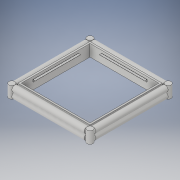
# Autodesk Inventor part: bumpers
Saved by Autodesk Inventor 2018 (Build 220112000, 112)
## iProperties
Created: 2019-02-23
Part Number: bumpers
Material: Generic
Document SubType Name: Modeling
Designer: s-2513226
Density: 1 g/cm^3
Appearance: Default
Author: s-2513226
Autodesk Inventor part; units mm, degrees
ref_plane "YZ Plane" through (0, 0, 0) normal (1, 0, 0) x (0, 1, 0)
ref_plane "XZ Plane" through (0, 0, 0) normal (0, 1, 0) x (-1, 0, 0)
ref_plane "XY Plane" through (0, 0, 0) normal (0, 0, 1) x (1, 0, 0)
sketch "Sketch1" plane through (0, 0, 0) normal (0, 0, 1) x (1, 0, 0)
  line L0 (0, 0) -> (-18.923, 0)
  line L1 (-18.923, 0) -> (-18.923, -127)
  line L2 (-18.923, -127) -> (0, -127)
  line L3 (0, -127) -> (0, 0)
  dimension "d0" = 127
  dimension "d1" = 18.923
  constraints: 8 end point, 2 parallel, 1 horizontal, 1 perpendicular
  measures "d0" distance of L0.end L1.end
  measures "d1" distance of L1.end L2.end
extrude "Extrusion1" add sketch "Sketch1" along normal blind 762
sketch "Sketch2" plane through (0, -127, 0) normal (1, 0, 0) x (0, 0, -1)
  line L0 (0, 127) -> (0, 0) projected
  line L1 (0, 127) -> (-18.923, 127)
  line L2 (-18.923, 127) -> (-18.923, 0)
  line L3 (-18.923, 0) -> (0, 0)
  line L4 (0, 0) -> (0, 127)
  dimension "d4" = 18.923
  dimension "d21" = 127
  constraints: 8 end point, 2 parallel, 1 horizontal, 1 perpendicular
  measures "d4" distance of L0.start L1.end
  measures "d21" distance of L3.end L0.start
extrude "Extrusion2" add sketch "Sketch2" along normal blind 762
sketch "Sketch3" plane through (0, -139.7, 18.923) normal (0, 0, 1) x (1, 0, 0)
  line L0 (762, 139.7) -> (-18.923, 139.7) projected
  line L1 (762, 139.7) -> (743.077, 139.7)
  line L2 (743.077, 139.7) -> (743.077, 12.7)
  line L3 (743.077, 12.7) -> (762, 12.7)
  line L4 (762, 12.7) -> (762, 139.7)
  line L5 (0, 12.7) -> (762, 12.7) projected
  point P0 (0, 139.7)
  dimension "d8" = 18.923
  constraints: 8 end point, 2 parallel, 1 horizontal, 1 perpendicular
  measures "d8" distance of L2.end L3.end
extrude "Extrusion3" add sketch "Sketch3" along normal blind 762
sketch "Sketch4" plane through (743.077, -127, 18.923) normal (-1, 0, 0) x (0, 0, 1)
  line L0 (762, 0) -> (762, 127) projected
  line L1 (762, 127) -> (743.077, 127)
  line L2 (743.077, 127) -> (743.077, 0)
  line L3 (743.077, 0) -> (762, 0)
  line L4 (762, 0) -> (762, 127)
  line L5 (0, 0) -> (762, 0) projected
  point P0 (-18.923, 127)
  dimension "d11" = 18.923
  dimension "d12" = 0
  constraints: 8 end point, 2 parallel, 1 horizontal, 1 perpendicular
  measures "d11" distance of L0.end L1.end
  measures "d12" distance between parallel lines of L5 L3
extrude "Extrusion4" add sketch "Sketch4" along normal blind 762
sketch "Sketch8" plane through (0, -139.7, 780.923) normal (0, 0, 1) x (1, 0, 0)
  circle A0 centre (-50.673, 107.95) radius 31.75
  circle A1 centre (-50.673, 44.45) radius 31.75
  line L0 (762, 12.7) -> (-18.923, 12.7) projected
  line L1 (762, 139.7) -> (-18.923, 139.7) projected
  line L2 (-18.923, 12.7) -> (-18.923, 139.7) projected
  point P0 (0, 139.7)
  dimension "d32" = 63.5
  dimension "d33" = 63.5
  dimension "d35" = 31.75
  dimension "d36" = 31.75
  dimension "d37" = 31.75
  dimension "d38" = 31.75
  constraints: 2 centre point
  measures "d32" diameter of A0
  measures "d33" diameter of A1
  measures "d35" distance from line of L1 A0.centre
  measures "d36" distance from line of L0 A1.centre
  measures "d37" distance from line of L2 A1.centre
  measures "d38" distance from line of L2 A0.centre
extrude "Extrusion7" add sketch "Sketch8" against normal blind 780.923 contours A0 | A1
sketch "Sketch10" plane through (-18.923, 0, 0) normal (-1, 0, 0) x (0, 0, 1)
  circle A0 centre (-31.75, -31.75) radius 31.75
  circle A1 centre (-31.75, -95.25) radius 31.75
  line L0 (0, 0) -> (0, -31.75) projected
  line L1 (0, 0) -> (780.923, 0) projected
  line L2 (0, 0) -> (0, -31.75) projected
  point P0 (0, -127)
  point P1 (0, -95.25)
  dimension "d41" = 63.5
  dimension "d42" = 63.5
  dimension "d43" = 31.75
  dimension "d44" = 31.75
  dimension "d45" = 31.75
  dimension "d46" = 31.75
  dimension "d47" = 31.75
  constraints: 2 centre point
  measures "d41" diameter of A0
  measures "d42" diameter of A1
  measures "d43" horizontal distance of point (0, -127) A1.centre
  measures "d44" horizontal distance of L0.start A0.centre
  measures "d45" distance from line of L0 A0.centre
  measures "d46" distance from line of L1 A0.centre
  measures "d47" distance from line of L2 A1.centre
extrude "Extrusion8" add sketch "Sketch10" against normal blind 780.923
sketch "Sketch12" plane through (0, 0, 0) normal (0, 0, -1) x (-1, 0, 0)
  circle A0 centre (-793.75, -31.75) radius 31.75
  circle A1 centre (-793.75, -95.25) radius 31.75
  line L0 (-762, -63.5) -> (-762, -127) projected
  line L1 (-762, 0) -> (-762, -63.5) projected
  line L2 (-762, 0) -> (18.923, 0) projected
  line L3 (18.923, -127) -> (-762, -127) projected
  point P0 (0, 0)
  point P1 (-762, -95.25)
  point P2 (-762, -31.75)
  dimension "d50" = 63.5
  dimension "d51" = 63.5
  dimension "d52" = 31.75
  dimension "d53" = 31.75
  dimension "d54" = 31.75
  dimension "d55" = 31.75
  constraints: 2 centre point
  measures "d50" diameter of A0
  measures "d51" diameter of A1
  measures "d52" distance from line of L0 A1.centre
  measures "d53" distance from line of L1 A0.centre
  measures "d54" distance from line of L2 A0.centre
  measures "d55" distance from line of L3 A1.centre
extrude "Extrusion9" add sketch "Sketch12" against normal blind 780.923 contours A0 | A1
sketch "Sketch13" plane through (762, -127, 0) normal (1, 0, 0) x (0, 0, -1)
  circle A0 centre (-812.673, 95.25) radius 31.75
  circle A1 centre (-812.673, 31.75) radius 31.75
  line L0 (0, 127) -> (-780.923, 127) projected
  line L1 (-780.923, 127) -> (-780.923, 63.5) projected
  line L2 (-780.923, 63.5) -> (-780.923, 0) projected
  point P0 (0, 0)
  point P1 (-762, -95.25)
  point P2 (-762, -31.75)
  point P3 (-780.923, 95.25)
  point P4 (-780.923, 31.75)
  dimension "d58" = 63.5
  dimension "d59" = 63.5
  dimension "d64" = 63.5
  dimension "d65" = 31.75
  dimension "d66" = 31.75
  dimension "d67" = 31.75
  constraints: 2 centre point
  measures "d58" diameter of A0
  measures "d59" diameter of A1
  measures "d64" distance of A1.centre A0.centre
  measures "d65" distance from line of L0 A0.centre
  measures "d66" distance from line of L1 A0.centre
  measures "d67" distance from line of L2 A1.centre
extrude "Extrusion10" add sketch "Sketch13" against normal blind 780.923 contours A0 | A1
sketch "Sketch14" plane through (-18.923, 0, 0) normal (0, 1, 0) x (1, 0, 0)
  line L0 (780.923, 0) -> (812.673, 0) projected
  circle A0 centre (812.673, 31.75) radius 31.75
  line L1 (780.923, 0) -> (844.423, 0) projected
  line L2 (780.923, 0) -> (780.923, 63.5) projected
  circle A1 centre (-31.75, 31.75) radius 31.75
  line L3 (0, 0) -> (0, 63.5) projected
  line L4 (0, 0) -> (-63.5, 0) projected
  circle A2 centre (-31.75, -812.673) radius 31.75
  line L5 (0, -780.923) -> (-63.5, -780.923) projected
  line L6 (0, -780.923) -> (0, -844.423) projected
  circle A3 centre (812.673, -812.673) radius 31.75
  line L7 (780.923, -780.923) -> (844.423, -780.923) projected
  line L8 (780.923, -780.923) -> (780.923, -844.423) projected
  point P0 (18.923, 0)
  point P1 (780.923, 31.75)
  point P2 (0, 31.75)
  point P3 (-31.75, 0)
  point P4 (-31.75, -780.923)
  point P5 (0, -812.673)
  point P6 (812.673, -780.923)
  point P7 (780.923, -812.673)
  dimension "d73" = 63.5
  dimension "d76" = 63.5
  dimension "d70" = 31.75
  dimension "d71" = 63.5
  dimension "d72" = 31.75
  dimension "d74" = 31.75
  dimension "d75" = 31.75
  dimension "d77" = 31.75
  dimension "d78" = 31.75
  dimension "d79" = 63.5
  dimension "d80" = 31.75
  dimension "d81" = 31.75
  constraints: 2 centre point, 1 horizontal alignment, 1 point on circle, 1 vertical alignment, 2 other
  measures "d70" distance from line of L1 A0.centre
  measures "d71" diameter of A0
  measures "d72" distance from line of L2 A0.centre
  measures "d74" distance from line of point (-31.75, 31.75) L3
  measures "d75" distance from line of L4 point (-31.75, 31.75)
  measures "d77" distance from line of L5 point (-31.75, -812.673)
  measures "d78" distance from line of point (-31.75, -812.673) L6
  measures "d79" diameter of A3
  measures "d80" distance from line of L7 A3.centre
  measures "d81" distance from line of L8 A3.centre
extrude "Extrusion11" add sketch "Sketch14" against normal blind 127 contours A0 | A1 | A2 | A3
sketch "Sketch15" plane through (0, -127, 18.923) normal (1, 0, 0) x (0, 0, -1)
  line L0 (0, 0) -> (0, 127) projected
  line L1 (-743.077, 0) -> (-743.077, 127) projected
  line L2 (0, 0) -> (-743.077, 0) projected
  line L3 (18.923, 0) -> (-762, 0) projected
  line L4 (-616.077, 73.66) -> (-127, 73.66)
  line L5 (-127, 73.66) -> (-127, 99.06)
  line L6 (-127, 99.06) -> (-616.077, 99.06)
  line L7 (-616.077, 99.06) -> (-616.077, 73.66)
  point P0 (18.923, 127)
  point P1 (-127, 0)
  point P2 (-590.677, 0)
  point P3 (-152.4, 0)
  point P4 (-336.677, 0)
  point P5 (-762, 0)
  dimension "d99" = 25.4
  dimension "d100" = 73.66
  dimension "d101" = 127
  dimension "d102" = 127
  constraints: 8 end point, 2 parallel, 1 horizontal, 1 perpendicular, 4 other
  measures "d99" distance of L6.end L4.start
  measures "d100" distance of the line from the sketch origin of L4
  measures "d101" distance between parallel lines of L1 L7
  measures "d102" distance between parallel lines of L0 L5
extrude "Extrusion15" add sketch "Sketch15" along normal blind 1.651
sketch "Sketch17" plane through (1.651, -127, 18.923) normal (1, 0, 0) x (0, 0, -1)
  line L0 (-127, 99.06) -> (-616.077, 99.06) projected
  line L1 (-127, 99.06) -> (-127, 73.66) projected
  line L2 (-616.077, 99.06) -> (-127, 99.06)
  line L3 (-127, 99.06) -> (-127, 97.409)
  line L4 (-127, 97.409) -> (-616.077, 97.409)
  line L5 (-616.077, 97.409) -> (-616.077, 99.06)
  point P0 (18.923, 127)
  dimension "d105" = 1.651
  constraints: 8 end point, 2 parallel, 1 horizontal, 1 perpendicular, 1 point on line
  measures "d105" distance of L2.end L3.end
extrude "Extrusion16" add sketch "Sketch17" along normal blind 23.749
sketch "Sketch20" plane through (743.077, -127, 762) normal (0, 0, -1) x (-1, 0, 0)
  line L0 (127, 73.66) -> (616.077, 73.66)
  line L1 (616.077, 73.66) -> (616.077, 99.06)
  line L2 (616.077, 99.06) -> (127, 99.06)
  line L3 (127, 99.06) -> (127, 73.66)
  line L4 (0, 0) -> (743.077, 0) projected
  line L5 (743.077, 0) -> (743.077, 127) projected
  line L6 (0, 0) -> (0, 127) projected
  dimension "d115" = 25.4
  dimension "d116" = 73.66
  dimension "d117" = 127
  dimension "d118" = 489.077
  dimension "d119" = 127
  constraints: 8 end point, 2 parallel, 1 horizontal, 1 perpendicular
  measures "d115" distance of L2.end L0.start
  measures "d116" distance between parallel lines of L4 L0
  measures "d117" distance between parallel lines of L5 L1
  measures "d118" distance of L1.end L2.end
  measures "d119" distance between parallel lines of L6 L3
extrude "Extrusion19" add sketch "Sketch20" along normal blind 1.651
sketch "Sketch21" plane through (743.077, -127, 18.923) normal (-1, 0, 0) x (0, 0, 1)
  line L0 (127, 73.66) -> (616.077, 73.66)
  line L1 (616.077, 73.66) -> (616.077, 99.06)
  line L2 (616.077, 99.06) -> (127, 99.06)
  line L3 (127, 99.06) -> (127, 73.66)
  line L4 (0, 0) -> (743.077, 0)
  line L5 (743.077, 0) -> (743.077, 127)
  line L6 (0, 0) -> (0, 127)
  dimension "d123" = 25.4
  dimension "d124" = 73.66
  dimension "d122" = 127
  dimension "d125" = 489.077
  dimension "d129" = 127
  constraints: 14 end point, 2 parallel, 1 horizontal, 1 perpendicular
  measures "d123" distance of L2.end L0.start
  measures "d124" distance between parallel lines of L4 L0
  measures "d122" distance between parallel lines of L5 L1
  measures "d125" distance of L1.end L2.end
  measures "d129" distance between parallel lines of L6 L3
extrude "Extrusion20" add sketch "Sketch21" along normal blind 1.651
sketch "Sketch22" plane through (0, -127, 18.923) normal (0, 0, 1) x (1, 0, 0)
  line L0 (127, 73.66) -> (616.077, 73.66)
  line L1 (616.077, 73.66) -> (616.077, 99.06)
  line L2 (616.077, 99.06) -> (127, 99.06)
  line L3 (127, 99.06) -> (127, 73.66)
  line L4 (0, 0) -> (743.077, 0)
  line L5 (743.077, 0) -> (743.077, 127)
  line L6 (0, 0) -> (0, 127)
  dimension "d131" = 25.4
  dimension "d132" = 73.66
  dimension "d130" = 127
  dimension "d133" = 489.077
  dimension "d137" = 127
  constraints: 14 end point, 2 parallel, 1 horizontal, 1 perpendicular
  measures "d131" distance of L2.end L0.start
  measures "d132" distance between parallel lines of L4 L0
  measures "d130" distance between parallel lines of L5 L1
  measures "d133" distance of L1.end L2.end
  measures "d137" distance between parallel lines of L6 L3
extrude "Extrusion21" add sketch "Sketch22" along normal blind 1.651
sketch "Sketch23" plane through (0, -127, 20.574) normal (0, 0, 1) x (1, 0, 0)
  line L0 (616.077, 99.06) -> (127, 99.06) projected
  line L1 (616.077, 99.06) -> (127, 99.06)
  line L2 (127, 99.06) -> (127, 97.409)
  line L3 (127, 97.409) -> (616.077, 97.409)
  line L4 (616.077, 97.409) -> (616.077, 99.06)
  point P0 (0, 127)
  dimension "d138" = 1.651
  constraints: 8 end point, 2 parallel, 1 horizontal, 1 perpendicular
  measures "d138" distance of L1.end L2.end
extrude "Extrusion22" add sketch "Sketch23" along normal blind 23.749
sketch "Sketch24" plane through (743.077, -127, 760.349) normal (0, 0, -1) x (-1, 0, 0)
  line L0 (127, 99.06) -> (616.077, 99.06)
  line L1 (616.077, 99.06) -> (616.077, 97.409)
  line L2 (616.077, 97.409) -> (127, 97.409)
  line L3 (127, 97.409) -> (127, 99.06)
  point P0 (743.077, 127)
  dimension "d141" = 1.651
  constraints: 8 end point, 2 parallel, 1 horizontal, 1 perpendicular
  measures "d141" distance of L0.end L1.end
extrude "Extrusion23" add sketch "Sketch24" along normal blind 23.749
sketch "Sketch26" plane through (741.426, -127, 18.923) normal (-1, 0, 0) x (0, 0, 1)
  line L0 (127, 73.66) -> (127, 99.06) projected
  line L1 (616.077, 99.06) -> (616.077, 73.66) projected
  line L2 (127, 99.06) -> (616.077, 99.06)
  line L3 (616.077, 99.06) -> (616.077, 97.409)
  line L4 (616.077, 97.409) -> (127, 97.409)
  line L5 (127, 97.409) -> (127, 99.06)
  point P0 (-18.923, 127)
  dimension "d144" = 1.651
  constraints: 8 end point, 2 parallel, 1 horizontal, 1 perpendicular, 1 point on line
  measures "d144" distance of L2.end L3.end
extrude "Extrusion24" add sketch "Sketch26" along normal blind 23.749
body "Solid1"
